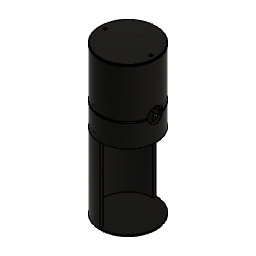
Freshener_Dispenser_Case (Autodesk Fusion 360 design; units mm, degrees)
Autodesk Fusion 360 part; units mm, degrees
note: some values were not read from the file. Chosen so that the rebuilt part matches the saved one: which face or edge a step refers to; which bodies a step acts on; which pieces of a blend or face edit are solid. Set by a fixed rule: which sketch regions a step uses.
(part 1 of 2)
sketch "Sketch1" plane through (0, 0, 0) normal (0, 0, 1) x (1, 0, 0)
  circle A0 centre (0, 0) radius 37.5
  dimension "d1" = 75
  constraint coincident A0.centre origin
  measures "d1" diameter of A0
extrude "Extrude1" add sketch "Sketch1" along normal blind 2 makes body 1
sketch "Sketch2" plane through (0, 0, 2) normal (0, 0, 1) x (-1, 0, 0)
  circle A0 centre (0, 0) radius 37.5
  circle A1 centre (0, 0) radius 33.5
  dimension "d4" = 67
  constraint coincident A0.centre A1.centre
  measures "d4" diameter of A1
extrude "Extrude2" add sketch "Sketch2" along normal blind 196 bodies 1
move_body "Move1" bodies 1 to x (0, 1, 0) y (-1, 0, 0) z (0, 0, 1) at (-0.5, -0.5, 0)
ref_plane "WorkPlane2" through (37, 0, 0) normal (1, 0, 0) x (0, 1, 0)
sketch "Sketch4" plane through (37, 0, 0) normal (1, 0, 0) x (0, 1, 0)
  line L0 (37.676, 2) -> (-39.4371, 2)
  line L1 (-39.4371, 2) -> (-39.4371, 102)
  line L2 (-39.4371, 102) -> (37.676, 102)
  line L3 (37.676, 102) -> (37.676, 2)
  line L4 (37, 0) -> (-38, 0)
  dimension "d14" = 100
  dimension "d15" = 2
  constraint horizontal L0
  constraint vertical L1
  constraint horizontal L2
  constraint vertical L3
  measures "d14" distance of L0.start L2.end
  measures "d15" distance of L0 L4
extrude "Extrude4" cut sketch "Sketch4" against normal blind 37.5 bodies 1
move_body "Move2" bodies 1 to x (1, 0, 0) y (0, 1, 0) z (0, 0, 1) at (0, 0.5, 0)
move_body "Move3" bodies 1 to x (1, 0, 0) y (0, 1, 0) z (0, 0, 1) at (0.5, 0, 0)
sketch "Sketch7" plane through (37, 0, 0) normal (1, 0, 0) x (0, 1, 0)
  circle A0 centre (0, 134) radius 0.25
  circle A1 through (10, 134, 1) (-5, 142.6603, 1) (-5, 125.3397, 1)
  dimension "d33" = 20
sketch "Sketch7 (curves 1 mm off its plane)" plane through (38, 0, 0) normal (1, 0, 0) x (0, 1, 0)
  circle A0 centre (0, 134) radius 10
extrude "Extrude6" cut sketch "Sketch7 (curves 1 mm off its plane)" against normal blind 6 bodies 1
ref_plane "WorkPlane3" through (0, 0, 133.75) normal (0, 0, 1) x (1, 0, 0)
sketch "Sketch6" plane through (0, 0, 133.75) normal (0, 0, 1) x (1, 0, 0)
  circle A0 centre (0, 0) radius 37.5
  spline S0 degree 3 poles (36.345, -9.2353) (36.345, -9.2353) (36.4749, -8.7241) (36.6575, -7.9556) (36.9971, -6.1867) (37.1768, -5.0663) (37.4299, -2.6043) (37.5, -1.2621) (37.5, 1.2621) (37.4299, 2.6043) (37.1768, 5.0663) (36.9971, 6.1867) (36.6575, 7.9556) (36.4749, 8.7241) (36.2151, 9.7465) (36.1421, 10) (36.1421, 10) knots 0 0.378704 0.378704 0.378704 0.378704 0.757408 0.757408 1.136043 1.136043 1.514678 1.514678 1.893313 1.893313 2.271948 2.271948 2.650652 2.650652 3.029356 3.029356 3.029356 3.029356
  line L0 (0, -7) -> (-17, -7)
  line L1 (-17, -7) -> (-17, 7)
  line L2 (-17, 7) -> (0, 7)
  line L3 (36.1439, -9.9936) -> (0, -7)
  line L4 (36.1421, 10) -> (0, 7)
  dimension "d47" = 75
  constraint coincident A0.centre origin
  constraint horizontal L0
  constraint perpendicular L0 L1
  constraint perpendicular L1 L2
  constraint coincident S0.end L4.start
  constraint coincident A0 L3.start
  measures "d47" diameter of A0
extrude "Extrude10" add sketch "Sketch6" against normal blind 2 separate body makes body 2
extrude "Extrude7" cut sketch "Sketch6" against normal blind 2 contours A0 L0 L1 L2 L3 L4 picked at (12.5, 0) bodies 1 2
sketch "Sketch9" plane through (0, 0, 133.75) normal (0, 0, -1) x (-1, 0, 0)
  line L0 (2.5299, 20.125) -> (-2.4701, 20.125)
  line L1 (-2.4701, 20.125) -> (-2.4701, 17.375)
  line L2 (-2.4701, 17.375) -> (2.5299, 17.375)
  line L3 (2.5299, 17.375) -> (2.5299, 20.125)
  line L4 (-2.6701, 17.175) -> (2.7299, 17.175)
  line L5 (2.7299, 17.175) -> (2.7299, 20.325)
  line L6 (2.7299, 20.325) -> (-2.6701, 20.325)
  line L7 (-2.6701, 20.325) -> (-2.6701, 17.175)
  point P0 (-2.4701, 17.375)
  point P1 (2.5299, 17.375)
  point P2 (-2.4701, 20.125)
  point P3 (2.5299, 20.125)
  point P4 (0.0299, 18.75)
  dimension "d43" = 0.2
  constraint coincident P3 L0.start
  constraint coincident P2 L0.end
  constraint coincident P0 L1.end
  constraint coincident P1 L2.end
extrude "Extrude9" cut sketch "Sketch9" along normal blind 5 contours L0 L1 L2 L3 | L4 L5 L6 L7 bodies 1 2
ref_plane "WorkPlane4" through (0, 0, 102) normal (0, 0, 1) x (1, 0, 0)
split "Split1" by plane through (0, 0, 102) normal (0, 0, 1) bodies 1 makes body 3 at (1.8692, 37.4534, 134)
sketch "Sketch10" plane through (0, 0, 102) normal (0, 0, 1) x (-1, 0, 0)
  arc A0 (0, -37.5) -> (0, 37.5) centre (0, 0) ccw
  line L0 (0, 37.5) -> (0, 33.5)
  arc A1 (0, -33.5) -> (0, 33.5) centre (0, 0) ccw
  line L1 (0, -33.5) -> (0, -37.5)
  arc A2 (1.1, -34.5825) -> (1.1, 34.5825) centre (0, 0) ccw
  line L2 (1.1, 36.3834) -> (1.1, 34.5825)
  arc A3 (1.1, -36.3834) -> (1.1, 36.3834) centre (0, 0) ccw
  line L3 (1.1, -34.5825) -> (1.1, -36.3834)
  line L4 (1.3, -34.5756) -> (1.3, -36.3768)
  line L5 (1.3, 36.4) -> (1.3, 34.5756)
  dimension "d90" = 0.2
  dimension "d91" = 0.2
  constraint coincident A2 L4.start
  constraint coincident A3 L4.end
  constraint vertical L4
  constraint vertical L5
  constraint coincident A2 L5.end
  constraint concentric A1 A2
  constraint concentric A0 A3
  measures "d90" distance of L3 L4
  measures "d91" distance of L2 L5
extrude "Extrude11" add sketch "Sketch10" along normal blind 5 contours A2 A3 L4 L5 bodies 1
sketch "Sketch11" plane through (0, 0, 102) normal (0, 0, -1) x (1, 0, 0)
  circle A0 centre (0, 0) radius 33.5
  circle A1 centre (0, 0) radius 37.5
  circle A2 centre (0, 0) radius 36.6
  circle A3 centre (0, 0) radius 34.4
  line L0 (0, 34.4) -> (0, 36.6)
  line L1 (0, -34.4) -> (0, -36.6)
  dimension "d53" = -0.9
  dimension "d54" = 0.9
  constraint coincident A3 L0.start
  constraint coincident A2 L0.end
  constraint vertical L0
  constraint coincident A3 L1.start
  constraint coincident A2 L1.end
  constraint parallel L0 L1
extrude "Extrude12" cut sketch "Sketch11" against normal blind 5.4 contours A2 A3 L0 L1 picked at (-1.8183, -35.7304) bodies 3
ref_plane "WorkPlane5" through (0, 0, 131.75) normal (0, 0, 1) x (1, 0, 0)
split "Split2" by plane through (0, 0, 131.75) normal (0, 0, 1) bodies 3 makes body 4 at (35.2064, 12.9134, 155.3434)
ref_plane "WorkPlane6" through (0, 0, 133.75) normal (0, 0, 1) x (1, 0, 0)
split "Split3" by plane through (0, 0, 133.75) normal (0, 0, 1) bodies 4 makes body 5 at (35.2408, -12.8194, 156.2088)
delete_body "RemoveBody1" bodies 4
sketch "Sketch12" plane through (0, 0, 131.75) normal (0, 0, 1) x (-1, 0, 0)
  line L0 (-32.0517, -9.7436) -> (-36.212, -9.7436)
  arc A0 (-36.212, -9.7436) -> (-36.212, 9.7436) centre (0, 0) ccw
  line L1 (-36.212, 9.7436) -> (-32.0517, 9.7436)
  arc A1 (-32.0517, -9.7436) -> (-32.0517, 9.7436) centre (0, 0) ccw
  arc A2 (-32.8569, -10.8436) -> (-32.8569, 10.8436) centre (0, 0) ccw
  line L2 (-34.7473, 10.8436) -> (-32.8569, 10.8436)
  arc A3 (-34.7473, -10.8436) -> (-34.7473, 10.8436) centre (0, 0) ccw
  line L3 (-32.8569, -10.8436) -> (-34.7473, -10.8436)
  line L4 (36.4, 0) -> (34.6, 0)
  line L5 (-0.0001, -34.6) -> (-0.0001, -36.4)
  line L6 (-0.0001, 36.4) -> (-0.0001, 34.6)
  line L7 (0, 0) -> (25.7387, -25.7387)
  line L8 (0, 0) -> (36.6, 0) construction
  line L9 (0, 0) -> (25.7387, 25.7387)
  line L10 (0, 0) -> (36.6, 0) construction
  line L11 (0, 0) -> (33.6292, -13.9297)
  line L12 (0, 0) -> (36.6, 0) construction
  line L13 (0, 0) -> (33.6292, 13.9297)
  line L14 (0, 0) -> (13.9297, 33.6292)
  line L15 (0, 0) -> (13.9297, -33.6292)
  line L16 (0, 0) -> (36.6, 0) construction
  line L17 (0, 0) -> (-13.9297, 33.6292)
  line L18 (0, 0) -> (36.6, 0) construction
  line L19 (0, 0) -> (-13.9297, -33.6292)
  line L20 (0, 0) -> (-25.8801, -25.8801)
  line L21 (0, 0) -> (36.6, 0) construction
  line L22 (-34.6843, -11.0436) -> (-32.7902, -11.0436)
  line L23 (-25.8797, -25.5969) -> (-24.6069, -24.3241)
  line L24 (13.7447, -33.7052) -> (13.0558, -32.0422)
  line L25 (-13.7387, -33.6908) -> (-13.0558, -32.0422)
  line L26 (33.5522, -14.1142) -> (31.8892, -13.4254)
  line L27 (25.8797, -25.5969) -> (24.6069, -24.3241)
  line L28 (-13.7387, -33.6908) -> (-13.7447, -33.7052)
  dimension "d60" = 45
  dimension "d61" = 45
  dimension "d62" = 22.5
  dimension "d65" = 135
  dimension "d66" = 67.5
  dimension "d67" = 112.5
  dimension "d68" = 45
  dimension "d69" = 135
  dimension "d80" = 0.2
  dimension "d81" = 0.2
  dimension "d82" = 0.2
  dimension "d83" = 0.2
  dimension "d84" = 0.2
  dimension "d85" = 0.2
  constraint midpoint A3 L4.start
  constraint midpoint A2 L4.end
  constraint coincident A2 L5.start
  constraint coincident A3 L5.end
  constraint perpendicular L4 L5
  constraint coincident A3 L6.start
  constraint coincident A2 L6.end
  constraint parallel L5 L6
  constraint horizontal L8
  constraint coincident A0.centre A1.centre
  constraint coincident A3 L7.end
  constraint horizontal L10
  constraint coincident A3 L9.end
  constraint horizontal L12
  constraint coincident A3 L11.end
  constraint coincident A3 L13.end
  constraint coincident A3 L14.end
  constraint horizontal L16
  constraint perpendicular L13 L15
  constraint horizontal L18
  constraint coincident A3 L17.end
  constraint coincident A3 L19.end
  constraint horizontal L21
  constraint coincident A3 L15.end
  constraint coincident A3 L22.start
  constraint coincident A2 L22.end
  constraint parallel L3 L22
  constraint coincident A3 L23.start
  constraint coincident A2 L23.end
  constraint parallel L20 L23
  constraint coincident A3 L24.start
  constraint coincident A2 L24.end
  constraint parallel L15 L24
  constraint coincident A2 L25.end
  constraint parallel L19 L25
  constraint coincident A3 L26.start
  constraint coincident A2 L26.end
  constraint parallel L11 L26
  constraint coincident A3 L27.start
  constraint coincident A2 L27.end
  constraint parallel L7 L27
  constraint coincident A3 L28.end
  constraint parallel L25 L28
  constraint concentric A1 A2
  constraint concentric A0 A3
  measures "d60" angle of L7 L8
  measures "d61" angle of L9 L10
  measures "d62" angle of L11 L12
  measures "d65" angle of L13 L14
  measures "d66" angle of L15 L16
  measures "d67" angle of L17 L18
  measures "d68" angle of L17 L19
  measures "d69" angle of L20 L21
  measures "d80" distance of L3 L22
  measures "d81" distance of L20 L23
  measures "d82" distance of L19 L25
  measures "d83" distance of L15 L24
  measures "d84" distance of L11 L26
  measures "d85" distance of L7 L27
extrude "Extrude13" add sketch "Sketch12" along normal blind 7 contours A2 A3 L22 L23 | A2 A3 L5 L25 L28 | A2 A3 L5 L24 | A2 A3 L26 L27 bodies 3
mirror "Mirror1" about plane through (0, 0, 0) normal (0, 1, 0) of "Extrude13"
sketch "Sketch13" plane through (0, 0, 133.75) normal (0, 0, 1) x (-1, 0, 0)
  line L0 (2.7299, -20.325) -> (-2.6701, -20.325)
  line L1 (-2.6701, -20.325) -> (-2.6701, -17.175)
  line L2 (-2.6701, -17.175) -> (2.7299, -17.175)
  line L3 (2.7299, -17.175) -> (2.7299, -20.325)
  line L4 (0, -7) -> (-36.1421, -10)
  arc A0 (-36.1421, -10) -> (-36.1439, 9.9936) centre (0, 0) ccw
  line L5 (-36.1439, 9.9936) -> (0, 7)
  line L6 (0, 7) -> (17, 7)
  line L7 (17, 7) -> (17, -7)
  line L8 (17, -7) -> (0, -7)
  line L9 (0.0372, 7.9) -> (17.9, 7.9)
  line L10 (17.9, 7.9) -> (17.9, -7.9)
  line L11 (17.9, -7.9) -> (0.0373, -7.9)
  line L12 (0.0373, -7.9) -> (-34.9685, -10.8057)
  arc A1 (-34.9685, -10.8057) -> (-34.9704, 10.7995) centre (0, 0) ccw
  line L13 (-34.9704, 10.7995) -> (0.0372, 7.9)
  arc A2 (-33.1543, -9.1733) -> (-33.156, 9.1675) centre (0, 0) ccw
  line L14 (13.9297, 33.6292) -> (13.2408, 31.9662)
  line L15 (-13.2408, 31.9662) -> (-13.9297, 33.6292)
  line L16 (-25.7387, 25.7387) -> (-24.4659, 24.4659)
  line L17 (-32.8569, 10.8436) -> (-34.7473, 10.8436)
  line L18 (24.4659, 24.4659) -> (25.7387, 25.7387)
  line L19 (33.6292, 13.9297) -> (31.9662, 13.2408)
  line L20 (-32.8569, 10.8436) -> (-32.6462, 10.8436)
  line L21 (-34.7473, 10.8436) -> (-34.9568, 10.8436)
  line L22 (-25.7387, 25.7387) -> (-25.8801, 25.8801)
  line L23 (-24.4659, 24.4659) -> (-24.3245, 24.3245)
  line L24 (-13.9297, 33.6292) -> (-14.0062, 33.814)
  line L25 (-13.2408, 31.9662) -> (-13.1643, 31.7815)
  line L26 (13.9297, 33.6292) -> (14.0062, 33.814)
  line L27 (13.2408, 31.9662) -> (13.1643, 31.7815)
  line L28 (25.7387, 25.7387) -> (25.8801, 25.8801)
  line L29 (24.4659, 24.4659) -> (24.3245, 24.3245)
  line L30 (33.6292, 13.9297) -> (33.814, 14.0062)
  line L31 (31.9662, 13.2408) -> (31.7815, 13.1643)
  dimension "d75" = -3.1
  constraint coincident L17.start L20.start
  constraint coincident A2 L20.end
  constraint parallel L17 L20
  constraint coincident L17.end L21.start
  constraint coincident A1 L21.end
  constraint horizontal L21
  constraint coincident L16.start L22.start
  constraint coincident A1 L22.end
  constraint parallel L16 L22
  constraint coincident L16.end L23.start
  constraint coincident A2 L23.end
  constraint parallel L16 L23
  constraint coincident L15.end L24.start
  constraint coincident A1 L24.end
  constraint parallel L15 L24
  constraint coincident L15.start L25.start
  constraint coincident A2 L25.end
  constraint parallel L15 L25
  constraint coincident L14.start L26.start
  constraint coincident A1 L26.end
  constraint parallel L14 L26
  constraint coincident L14.end L27.start
  constraint coincident A2 L27.end
  constraint parallel L14 L27
  constraint coincident L18.end L28.start
  constraint coincident A1 L28.end
  constraint parallel L18 L28
  constraint coincident L18.start L29.start
  constraint coincident A2 L29.end
  constraint parallel L18 L29
  constraint coincident L19.start L30.start
  constraint coincident A1 L30.end
  constraint parallel L19 L30
  constraint coincident L19.end L31.start
  constraint coincident A2 L31.end
  constraint parallel L19 L31
  constraint concentric A0 A1
extrude "Extrude14" cut sketch "Sketch13" against normal blind 2 contours A1 A2 L18 L19 L28 L29 L30 L31 | A1 A2 L14 L15 L24 L25 L26 L27 | A1 A2 L16 L17 L20 L21 L22 L23 bodies 2
mirror "Mirror2" about plane through (0, 0, 0) normal (0, 1, 0) of "Extrude14"
sketch "Sketch14" plane through (0, 0, 133.75) normal (0, 0, -1) x (1, 0, 0)
  line L0 (36.1429, -9.9969) -> (32, -9.9969)
  line L1 (32, -9.9969) -> (32, -9.9121)
  arc A0 (32, 9.9121) -> (32, -9.9121) centre (0, 0) ccw
  line L2 (32, 9.9121) -> (32, 9.9969)
  line L3 (32, 9.9969) -> (36.1429, 9.9969)
  arc A1 (36.1429, 9.9969) -> (36.1429, -9.9969) centre (0, 0) ccw
  line L4 (32.6462, 10.8436) -> (34.9568, 10.8436)
  arc A2 (32.6462, 10.8436) -> (24.3245, 24.3245) centre (0, 0) ccw
  arc A3 (34.9568, 10.8436) -> (25.8801, 25.8801) centre (0, 0) ccw
  line L5 (25.8801, 25.8801) -> (24.3245, 24.3245)
  arc A4 (13.1643, 31.7815) -> (-13.1643, 31.7815) centre (0, 0) ccw
  arc A5 (14.0062, 33.814) -> (-14.0062, 33.814) centre (0, 0) ccw
  line L6 (-14.0062, 33.814) -> (-13.1643, 31.7815)
  line L7 (13.1643, 31.7815) -> (14.0062, 33.814)
  line L8 (-33.814, 14.0062) -> (-31.7815, 13.1643)
  arc A6 (-25.8801, 25.8801) -> (-33.814, 14.0062) centre (0, 0) ccw
  arc A7 (-24.3245, 24.3245) -> (-31.7815, 13.1643) centre (0, 0) ccw
  line L9 (-24.3245, 24.3245) -> (-25.8801, 25.8801)
extrude "Extrude15" cut sketch "Sketch14" against normal blind 5.4 contours L4 A2 A3 L5 | A4 A5 L6 L7 | L8 A6 A7 L9 bodies 5
mirror "Mirror3" about plane through (0, 0, 0) normal (0, 1, 0) of "Extrude15"
sketch "Sketch15" plane through (0, 0, 198) normal (0, 0, 1) x (-1, 0, 0)
  circle A0 centre (0, 0) radius 33.5
  circle A1 centre (0, 0) radius 37.5
extrude "Extrude16" add sketch "Sketch15" along normal blind 2 separate body contours A0 | A1 makes body 6
sketch "Sketch16" plane through (0, 0, 198) normal (0, 0, -1) x (1, 0, 0)
  circle A0 centre (0, 0) radius 37.5
  circle A1 centre (0.2201, -17) radius 0.75
  circle A2 centre (0.2201, -17) radius 1.25
  dimension "d94" = 0.5
extrude "Extrude17" cut sketch "Sketch16" against normal blind 1 contours A1 | A2 bodies 6
sketch "Sketch19" plane through (0, 0, 198) normal (0, 0, 1) x (-1, 0, 0)
  circle A0 centre (0, 0) radius 33.5
  circle A1 centre (0, 0) radius 37.5
  line L0 (33.1246, -5.0014) -> (28.1246, -5.0014)
  line L1 (28.1246, -5.0014) -> (28.1246, 4.9986)
  line L2 (28.1246, 4.9986) -> (33.125, 4.9986)
  line L3 (33.5, -0.0014) -> (28.1246, -0.0014)
  circle A2 centre (30.8123, -0.0014) radius 1.25
  dimension "d105" = 5
  dimension "d106" = 5
  dimension "d107" = 5
  dimension "d110" = 2.5
  constraint coincident A0 L0.start
  constraint horizontal L0
  constraint perpendicular L0 L1
  constraint coincident A0 L2.end
  constraint perpendicular L1 L2
  constraint coincident A0 L3.start
  constraint coincident L1 L3.end
  constraint perpendicular L1 L3
  constraint midpoint L3 A2.centre
  measures "d105" distance of L0.start L0.end
  measures "d106" distance of L0 L3
  measures "d107" distance of L2 L3
  measures "d110" diameter of A2
extrude "Extrude21" add sketch "Sketch19" against normal blind 3 contours A0 L1 L2 L3 A2 | A0 L0 L1 L3 A2 bodies 5
mirror "Mirror6" about plane through (0, 0, 0) normal (1, 0, 0) of "Extrude21"
sketch "Sketch20" plane through (0, 0, 198) normal (0, 0, -1) x (1, 0, 0)
  circle A0 centre (0.2201, -17) radius 1.25
  circle A1 centre (0, 0) radius 37.5
  circle A2 centre (-30.8123, -0.0014) radius 1.25
  circle A3 centre (-30.8123, -0.0014) radius 2
  dimension "d115" = 0.75
extrude "Extrude22" cut sketch "Sketch20" against normal blind 2 contours A2 | A3 bodies 6
mirror "Mirror7" about plane through (0, 0, 0) normal (1, 0, 0) of "Extrude22"
sketch "Sketch21" plane through (0, 0, 133.75) normal (0, 0, 1) x (-1, 0, 0)
  arc A0 (-14.0062, -33.814) -> (14.0062, -33.814) centre (0, 0) ccw
  line L0 (-14.0062, -33.814) -> (-13.1643, -31.7815)
  arc A1 (-13.1643, -31.7815) -> (13.1643, -31.7815) centre (0, 0) ccw
  line L1 (13.1643, -31.7815) -> (14.0062, -33.814)
  arc A2 (-34.9568, -10.8436) -> (-25.8801, -25.8801) centre (0, 0) ccw
  line L2 (-34.9568, -10.8436) -> (-32.6462, -10.8436)
  arc A3 (-32.6462, -10.8436) -> (-24.3245, -24.3245) centre (0, 0) ccw
  line L3 (-24.3245, -24.3245) -> (-25.8801, -25.8801)
  arc A4 (25.8801, -25.8801) -> (33.814, -14.0062) centre (0, 0) ccw
  line L4 (25.8801, -25.8801) -> (24.3245, -24.3245)
  arc A5 (24.3245, -24.3245) -> (31.7815, -13.1643) centre (0, 0) ccw
  line L5 (31.7815, -13.1643) -> (33.814, -14.0062)
  arc A6 (14.0062, 33.814) -> (-14.0062, 33.814) centre (0, 0) ccw
  line L6 (14.0062, 33.814) -> (13.1643, 31.7815)
  arc A7 (13.1643, 31.7815) -> (-13.1643, 31.7815) centre (0, 0) ccw
  line L7 (-13.1643, 31.7815) -> (-14.0062, 33.814)
  arc A8 (-25.8801, 25.8801) -> (-34.9568, 10.8436) centre (0, 0) ccw
  line L8 (-25.8801, 25.8801) -> (-24.3245, 24.3245)
  arc A9 (-24.3245, 24.3245) -> (-32.6462, 10.8436) centre (0, 0) ccw
  line L9 (-32.6462, 10.8436) -> (-34.9568, 10.8436)
  arc A10 (33.814, 14.0062) -> (25.8801, 25.8801) centre (0, 0) ccw
  line L10 (33.814, 14.0062) -> (31.7815, 13.1643)
  arc A11 (31.7815, 13.1643) -> (24.3245, 24.3245) centre (0, 0) ccw
  line L11 (24.3245, 24.3245) -> (25.8801, 25.8801)
  line L12 (2.7299, -20.325) -> (-2.6701, -20.325)
  line L13 (-2.6701, -20.325) -> (-2.6701, -17.175)
  line L14 (-2.6701, -17.175) -> (2.7299, -17.175)
  line L15 (2.7299, -17.175) -> (2.7299, -20.325)
  line L16 (0, -7) -> (-36.1421, -10)
  arc A12 (-36.1421, -10) -> (-36.1439, 9.9936) centre (0, 0) ccw
  line L17 (-36.1439, 9.9936) -> (0, 7)
  line L18 (0, 7) -> (17, 7)
  line L19 (17, 7) -> (17, -7)
  line L20 (17, -7) -> (0, -7)
  line L21 (-36.0448, 11.1895) -> (0.0496, 8.2)
  line L22 (0.0496, 8.2) -> (18.2, 8.2)
  line L23 (18.2, 8.2) -> (18.2, -8.2)
  line L24 (18.2, -8.2) -> (0.0497, -8.2)
  line L25 (0.0497, -8.2) -> (-36.0428, -11.1959)
  line L26 (-31.578, 9.6154) -> (-31.1283, 10.7823)
  spline S0 degree 3 poles (-32.0517, 9.7436) (-32.0896, 9.619) (-32.1408, 9.4481) (-32.3488, 8.7229) (-32.5544, 7.9547) (-32.936, 6.1877) (-33.1376, 5.0683) (-33.4214, 2.6067) (-33.5, 1.2638) (-33.5, -1.2638) (-33.4214, -2.6067) (-33.1376, -5.0683) (-32.936, -6.1877) (-32.5544, -7.9547) (-32.3488, -8.7229) (-32.1408, -9.4481) (-32.0896, -9.619) (-32.0517, -9.7436) knots 0.220731 0.220731 0.220731 0.220731 0.37925 0.37925 0.7585 0.7585 1.137639 1.137639 1.516778 1.516778 1.895917 1.895917 2.275056 2.275056 2.654306 2.654306 2.812825 2.812825 2.812825 2.812825
  line L27 (11.9299, -8.2) -> (11.9299, -7)
  line L28 (11.2799, -8) -> (11.2799, -26)
  line L29 (-11.8701, -9.1894) -> (-11.8701, -7.9853)
  line L30 (-11.2201, -8.25) -> (-11.2201, -13.9459)
  line L31 (-35.7961, -11.1754) -> (-36.1421, -10)
  line L32 (-31.2057, -10.7944) -> (-31.5517, -9.619)
  point P0 (-32.078, 9.6568)
  point P1 (11.2799, -8.2)
  point P2 (-11.2201, -9.1355)
  dimension "d120" = -1.2
  dimension "d121" = 0.5
  dimension "d124" = 0.65
  dimension "d125" = 0.65
  dimension "d126" = 0.5
  constraint coincident L17 L26.start
  constraint coincident L21 L26.end
  constraint coincident S0 P0
  constraint coincident L17 P0
  constraint coincident L24 L27.start
  constraint coincident L20 L27.end
  constraint perpendicular L20 L27
  constraint coincident L28 P1
  constraint coincident L24 P1
  constraint coincident L25 L29.start
  constraint coincident L16 L29.end
  constraint vertical L29
  constraint coincident L30 P2
  constraint coincident L25 P2
  constraint coincident L25 L31.start
  constraint coincident A12 L31.start
  constraint coincident L16.end A12.start
  constraint coincident L25 L32.start
  constraint coincident L16 L32.end
  constraint parallel L31 L32
  measures "d121" horizontal distance of L26.start P0
  measures "d124" distance of L27.start P1
  measures "d125" horizontal distance of L29.start P2
  measures "d126" distance of S0.end L32.end
extrude "Extrude23" add sketch "Sketch21" along normal blind 25 contours L16 L25 L29 L32 | L17 L18 L19 L20 L21 L22 L23 L24 L26 L27 bodies 2
sketch "Sketch22" plane through (0, 0, 158.75) normal (0, 0, 1) x (-1, 0, 0)
  line L0 (-31.578, 9.6154) -> (0, 7)
  line L1 (0, 7) -> (17, 7)
  line L2 (17, 7) -> (17, -7)
  line L3 (17, -7) -> (11.9299, -7)
  line L4 (11.9299, -7) -> (11.9299, -8.2)
  line L5 (11.9299, -8.2) -> (18.2, -8.2)
  line L6 (18.2, -8.2) -> (18.2, 8.2)
  line L7 (18.2, 8.2) -> (0.0496, 8.2)
  line L8 (0.0496, 8.2) -> (-31.1283, 10.7823)
  line L9 (-31.1283, 10.7823) -> (-31.578, 9.6154)
  line L10 (18.2, -8.2) -> (18.2, 8.2)
  line L11 (18.2, 8.2) -> (0.0496, 8.2)
  line L12 (-31.1283, 10.7823) -> (0.0496, 8.2)
  line L13 (18.2, -8.2) -> (11.9299, -8.2)
  line L14 (-31.2057, -10.7944) -> (-11.8701, -9.1894)
  spline S0 degree 5 poles (-31.2057, -10.7944) (-31.3407, -10.3619) (-31.5987, -9.4971) (-31.9499, -8.2001) (-32.3455, -6.4712) (-32.7107, -4.311) (-32.9348, -2.1517) (-33.0065, 0.0065) (-32.9195, 2.1636) (-32.6799, 4.3197) (-32.2993, 6.4748) (-31.8912, 8.1982) (-31.5306, 9.4904) (-31.2664, 10.3517) (-31.1283, 10.7823) knots 0 0 0 0 0 0 0.1 0.2 0.3 0.4 0.5 0.6 0.7 0.8 0.9 1 1 1 1 1 1
  line L15 (11.9299, -8.2) -> (11.9299, -7)
  line L16 (11.9299, -7) -> (-11.8701, -7)
  line L17 (-11.8701, -7) -> (-11.8701, -9.1894)
  point P0 (-31.2057, -10.7944)
  point P1 (-11.8701, -9.1894)
  point P2 (-32.9669, 0.0108)
  constraint coincident L5.end L6.start
  constraint coincident L6.end L7.start
  constraint coincident L7.end L8.start
  constraint coincident L8.end L9.start
  constraint coincident L4.end L5.start
  constraint coincident P0 L14.start
  constraint coincident P1 L14.end
  constraint coincident L3.end L4.start
  constraint perpendicular L15 L16
  constraint parallel L15 L17
extrude "Extrude24" add sketch "Sketch22" along normal blind 1.2 separate body contours L0 L1 L2 L3 L4 L5 L6 L7 L8 L10 L11 L12 L13 S0 L15 | L0 L1 L2 L3 L14 S0 L16 L17 makes body 7
sketch "Sketch23" plane through (0, 0, 159.95) normal (0, 0, 1) x (-1, 0, 0)
  line L0 (18.2, -8.2) -> (18.2, 8.2)
  line L1 (18.2, 8.2) -> (0.0496, 8.2)
  line L2 (0.0496, 8.2) -> (-31.1283, 10.7823)
  spline S0 degree 5 poles (-31.1283, 10.7823) (-31.2664, 10.3517) (-31.5306, 9.4904) (-31.8912, 8.1982) (-32.2993, 6.4748) (-32.6799, 4.3197) (-32.9195, 2.1636) (-33.0065, 0.0065) (-32.9348, -2.1517) (-32.7107, -4.311) (-32.3455, -6.4712) (-31.9499, -8.2001) (-31.5987, -9.4971) (-31.3407, -10.3619) (-31.2057, -10.7944) knots -1 -1 -1 -1 -1 -1 -0.9 -0.8 -0.7 -0.6 -0.5 -0.4 -0.3 -0.2 -0.1 0 0 0 0 0 0
  line L3 (-31.2057, -10.7944) -> (-11.8701, -9.1894)
  line L4 (-11.8701, -9.1894) -> (-11.8701, -7)
  line L5 (-11.8701, -7) -> (11.9299, -7)
  line L6 (11.9299, -7) -> (11.9299, -8.2)
  line L7 (11.9299, -8.2) -> (18.2, -8.2)
  line L8 (12.4345, 7.3206) -> (12.4345, 8.2)
  line L9 (10.437, 7.3206) -> (10.437, 8.2)
  line L10 (9.937, 7.3206) -> (9.937, 8.2)
  line L11 (9.937, 7.3206) -> (9.937, -5.3794)
  line L12 (9.937, -5.3794) -> (9.937, -6.831)
  line L13 (12.9345, -5.3794) -> (12.9345, 7.3206)
  line L14 (12.9345, 7.3206) -> (12.9345, 8.2)
  line L15 (9.937, -6.831) -> (9.937, -7)
  line L16 (-6.5642, -4.356) -> (-4.5642, -4.356)
  line L17 (-6.5642, -3.106) -> (-4.5642, -3.106)
  line L18 (-4.5642, -4.356) -> (-3.9392, -4.356)
  line L19 (-3.9392, -4.356) -> (-3.9392, -3.106)
  line L20 (-3.9392, -3.106) -> (-4.5642, -3.106)
  line L21 (-6.5642, -3.106) -> (-7.1892, -3.106)
  line L22 (-7.1892, -3.106) -> (-7.1892, -4.356)
  line L23 (-7.1892, -4.356) -> (-6.5642, -4.356)
  line L24 (-3.1892, -5.106) -> (-3.1892, -2.356)
  line L25 (-3.1892, -2.356) -> (-4.5642, -2.356)
  line L26 (-6.5642, -2.356) -> (-4.5642, -2.356)
  line L27 (-6.5642, -2.356) -> (-7.9392, -2.356)
  line L28 (-7.9392, -2.356) -> (-7.9392, -5.106)
  line L29 (-7.9392, -5.106) -> (-6.5642, -5.106)
  line L30 (-6.5642, -5.106) -> (-4.5642, -5.106)
  line L31 (-4.5642, -5.106) -> (-3.1892, -5.106)
  line L32 (7.6451, 4.4702) -> (7.6451, 8.2)
  line L33 (7.6451, 4.4702) -> (6.5189, 4.4702)
  line L34 (6.5189, 4.4702) -> (6.4807, 8.2)
  line L35 (5.7765, 3.7202) -> (5.7308, 8.1923)
  line L36 (8.3951, 3.7202) -> (5.7765, 3.7202)
  line L37 (8.3951, 3.7202) -> (8.3951, 8.2)
  line L38 (8.3951, 8.2) -> (7.6451, 8.2)
  line L39 (8.3951, 8.2) -> (7.6451, 8.2)
  line L40 (5.7308, 8.1923) -> (5.7308, 8.2)
  line L41 (6.4807, 8.2) -> (5.7308, 8.2)
  circle A0 centre (-28.0642, 7.769) radius 1.5
  circle A1 centre (-28.0642, -5.731) radius 1.5
  circle A2 centre (-28.0642, 7.769) radius 0.75
  circle A3 centre (-28.0642, -5.731) radius 0.75
  dimension "d132" = 0.75
  dimension "d133" = -0.75
  dimension "d136" = 1.5
  dimension "d137" = 1.5
  constraint coincident L1 L8.end
  constraint perpendicular L1 L8
  constraint coincident L1 L9.end
  constraint perpendicular L1 L9
  constraint coincident L5 L15.end
  constraint perpendicular L5 L15
  constraint horizontal L16
  constraint parallel L16 L17
  constraint parallel L16 L18
  constraint perpendicular L17 L19
  constraint perpendicular L19 L20
  constraint parallel L17 L21
  constraint perpendicular L16 L22
  constraint perpendicular L22 L23
  constraint coincident L1 L32.end
  constraint perpendicular L1 L32
  constraint perpendicular L32 L33
  constraint coincident L1 L34.end
  constraint perpendicular L32 L38
  constraint coincident L1 L40.end
  constraint perpendicular L1 L40
  constraint concentric A0 A2
  constraint concentric A1 A3
  measures "d136" diameter of A2
  measures "d137" diameter of A3
extrude "Extrude25" cut sketch "Sketch23" against normal blind 1.2 contours L0 L1 L5 L6 L7 L10 L11 L12 L15 bodies 7
extrude "Extrude26" cut sketch "Sketch23" against normal blind 1.2 contours L1 L32 L33 L34 L35 L36 L37 L38 L39 L40 L41 | L1 L32 L33 L34 | L16 L17 L18 L19 L20 L21 L22 L23 | L24 L25 L26 L27 L28 L29 L30 L31 | A2 | A3 bodies 7
sketch "Sketch24" plane through (0, 0, 133.75) normal (0, 0, 1) x (-1, 0, 0)
  line L0 (-31.2057, -10.7944) -> (-31.5517, -9.619)
  line L1 (-31.5517, -9.619) -> (-36.1421, -10)
  arc A0 (-36.1421, -10) -> (-36.1439, 9.9936) centre (0, 0) ccw
  line L2 (-36.1439, 9.9936) -> (-31.578, 9.6154)
  line L3 (-31.578, 9.6154) -> (-31.1283, 10.7823)
  line L4 (-31.1283, 10.7823) -> (0.0496, 8.2)
  line L5 (0.0496, 8.2) -> (18.2, 8.2)
  line L6 (18.2, 8.2) -> (18.2, -8.2)
  line L7 (18.2, -8.2) -> (11.9299, -8.2)
  line L8 (11.9299, -8.2) -> (11.9299, -7)
  line L9 (11.9299, -7) -> (0, -7)
  line L10 (0, -7) -> (-11.8701, -7.9853)
  line L11 (-11.8701, -7.9853) -> (-11.8701, -9.1894)
  line L12 (-11.8701, -9.1894) -> (-31.2057, -10.7944)
  arc A1 (-14.0062, -33.814) -> (14.0062, -33.814) centre (0, 0) ccw
  line L13 (-14.0062, -33.814) -> (-13.1643, -31.7815)
  arc A2 (-13.1643, -31.7815) -> (13.1643, -31.7815) centre (0, 0) ccw
  line L14 (13.1643, -31.7815) -> (14.0062, -33.814)
  arc A3 (-34.9568, -10.8436) -> (-25.8801, -25.8801) centre (0, 0) ccw
  line L15 (-34.9568, -10.8436) -> (-32.6462, -10.8436)
  arc A4 (-32.6462, -10.8436) -> (-24.3245, -24.3245) centre (0, 0) ccw
  line L16 (-24.3245, -24.3245) -> (-25.8801, -25.8801)
  arc A5 (25.8801, -25.8801) -> (33.814, -14.0062) centre (0, 0) ccw
  line L17 (25.8801, -25.8801) -> (24.3245, -24.3245)
  arc A6 (24.3245, -24.3245) -> (31.7815, -13.1643) centre (0, 0) ccw
  line L18 (31.7815, -13.1643) -> (33.814, -14.0062)
  arc A7 (14.0062, 33.814) -> (-14.0062, 33.814) centre (0, 0) ccw
  line L19 (14.0062, 33.814) -> (13.1643, 31.7815)
  arc A8 (13.1643, 31.7815) -> (-13.1643, 31.7815) centre (0, 0) ccw
  line L20 (-13.1643, 31.7815) -> (-14.0062, 33.814)
  arc A9 (-25.8801, 25.8801) -> (-34.9568, 10.8436) centre (0, 0) ccw
  line L21 (-25.8801, 25.8801) -> (-24.3245, 24.3245)
  arc A10 (-24.3245, 24.3245) -> (-32.6462, 10.8436) centre (0, 0) ccw
  line L22 (-32.6462, 10.8436) -> (-34.9568, 10.8436)
  arc A11 (33.814, 14.0062) -> (25.8801, 25.8801) centre (0, 0) ccw
  line L23 (33.814, 14.0062) -> (31.7815, 13.1643)
  arc A12 (31.7815, 13.1643) -> (24.3245, 24.3245) centre (0, 0) ccw
  line L24 (24.3245, 24.3245) -> (25.8801, 25.8801)
  line L25 (2.7299, -20.325) -> (-2.6701, -20.325)
  line L26 (-2.6701, -20.325) -> (-2.6701, -17.175)
  line L27 (-2.6701, -17.175) -> (2.7299, -17.175)
  line L28 (2.7299, -17.175) -> (2.7299, -20.325)
  circle A13 centre (20.8, 11.2) radius 1
  circle A14 centre (-20.5, 11.2) radius 1
  circle A15 centre (20.8, 11.2) radius 0.75
  circle A16 centre (-20.5, 11.2) radius 0.75
  ellipse E0 centre (-17.6329, 26.63) end of major axis (-17.6329, 25.7781) minor radius 0.8519
  ellipse E1 centre (17.9271, 26.63) end of major axis (17.9271, 25.7781) minor radius 0.8519
  line L29 (17.9271, 26.63) -> (-17.6329, 26.63)
  line L30 (17.9271, 26.63) -> (17.9271, 25.7781)
  line L31 (17.9271, 26.63) -> (17.9271, 27.4819)
  line L32 (17.9271, 25.7781) -> (-17.6329, 25.7781)
  line L33 (17.9271, 27.4819) -> (-17.6329, 27.4819)
  line L34 (17.9271, 26.63) -> (18.779, 26.63)
  line L35 (18.779, 26.63) -> (18.779, 25.7781)
  line L36 (18.779, 25.7781) -> (17.9271, 25.7781)
  line L37 (17.9271, 27.4819) -> (18.779, 27.4819)
  line L38 (18.779, 27.4819) -> (18.779, 26.63)
  line L39 (-17.6329, 26.63) -> (-18.4848, 26.63)
  line L40 (-18.4848, 26.63) -> (-18.4848, 25.7781)
  line L41 (-18.4848, 25.7781) -> (-17.6329, 25.7781)
  line L42 (-18.4848, 26.63) -> (-18.4848, 27.4819)
  line L43 (-18.4848, 27.4819) -> (-17.6329, 27.4819)
  line L44 (19.279, 26.63) -> (19.279, 25.2781)
  line L45 (19.279, 25.2781) -> (17.9271, 25.2781)
  line L46 (17.9271, 25.2781) -> (-17.6329, 25.2781)
  line L47 (-18.9848, 25.2781) -> (-17.6329, 25.2781)
  line L48 (-18.9848, 26.63) -> (-18.9848, 25.2781)
  line L49 (-18.9848, 26.63) -> (-18.9848, 27.9819)
  line L50 (-18.9848, 27.9819) -> (-17.6329, 27.9819)
  line L51 (17.9271, 27.9819) -> (-17.6329, 27.9819)
  line L52 (17.9271, 27.9819) -> (19.279, 27.9819)
  line L53 (19.279, 27.9819) -> (19.279, 26.63)
  dimension "d138" = 1.5
  dimension "d139" = 1.5
  dimension "d142" = -0.5
  constraint concentric A13 A15
  constraint concentric A14 A16
  constraint coincident E1.centre L29.start
  constraint coincident E0.centre L29.end
  constraint coincident E1 L30.end
  constraint perpendicular L29 L30
  constraint coincident E1 L31.end
  constraint perpendicular L29 L31
  constraint coincident E0 L32.end
  constraint perpendicular L30 L32
  constraint coincident E0 L33.end
  constraint tangent E1 L33
  constraint coincident E1 L34.end
  constraint parallel L29 L34
  constraint perpendicular L29 L35
  constraint perpendicular L35 L36
  constraint perpendicular L31 L37
  constraint perpendicular L37 L38
  constraint coincident E0 L39.end
  constraint perpendicular L38 L39
  constraint perpendicular L32 L40
  constraint perpendicular L40 L41
  constraint perpendicular L33 L42
  constraint perpendicular L42 L43
  measures "d138" diameter of A15
  measures "d139" diameter of A16
extrude "Extrude27" cut sketch "Sketch24" against normal blind 2 contours A15 | A16 bodies 2
extrude "Extrude28" add sketch "Sketch24" along normal blind 1.5 contours L44 L45 L46 L47 L48 L49 L50 L51 L52 L53 bodies 2
ref_plane "WorkPlane8" through (0, -33.5, 0) normal (0, 1, 0) x (0, 0, 1)
sketch "Sketch27" plane through (0, -33.5, 0) normal (0, 1, 0) x (1, 0, 0)
  circle A0 centre (8.8696, -178.6636) radius 1.75
  circle A1 centre (8.8696, -178.6636) radius 2.25
  dimension "d154" = 0.5
extrude "Extrude31" add sketch "Sketch27" along normal blind 3.25 contours A0 | A1 bodies 5
mirror "Mirror9" about plane through (0, 0, 0) normal (1, 0, 0) of "Extrude31"
sketch "Sketch28" plane through (0, -30.25, 0) normal (0, 1, 0) x (-1, 0, 0)
  circle A0 centre (-8.8696, 178.6636) radius 2.25
  circle A1 centre (-8.8696, 178.6636) radius 0.875
  dimension "d160" = 1.75
  constraint concentric A0 A1
  measures "d160" diameter of A1
extrude "Extrude32" cut sketch "Sketch28" against normal blind 4 contours A1 bodies 5
fillet "Fillet1" radius 0.5 2 edges at (13.5606, -34.9623, 0) (34.9623, 13.5606, 200) on bodies 1 6
sketch "Sketch29" plane through (0, 0, 133.75) normal (0, 0, 1) x (-1, 0, 0)
  line L0 (2.7299, -20.325) -> (-2.6701, -20.325)
  line L1 (-2.6701, -20.325) -> (-2.6701, -17.175)
  line L2 (-2.6701, -17.175) -> (2.7299, -17.175)
  line L3 (2.7299, -17.175) -> (2.7299, -20.325)
  arc A0 (33.814, 14.0062) -> (25.8801, 25.8801) centre (0, 0) ccw
  line L4 (33.814, 14.0062) -> (31.7815, 13.1643)
  arc A1 (31.7815, 13.1643) -> (24.3245, 24.3245) centre (0, 0) ccw
  line L5 (24.3245, 24.3245) -> (25.8801, 25.8801)
  arc A2 (-25.8801, 25.8801) -> (-34.9568, 10.8436) centre (0, 0) ccw
  line L6 (-25.8801, 25.8801) -> (-24.3245, 24.3245)
  arc A3 (-24.3245, 24.3245) -> (-32.6462, 10.8436) centre (0, 0) ccw
  line L7 (-32.6462, 10.8436) -> (-34.9568, 10.8436)
  arc A4 (14.0062, 33.814) -> (-14.0062, 33.814) centre (0, 0) ccw
  line L8 (14.0062, 33.814) -> (13.1643, 31.7815)
  arc A5 (13.1643, 31.7815) -> (-13.1643, 31.7815) centre (0, 0) ccw
  line L9 (-13.1643, 31.7815) -> (-14.0062, 33.814)
  arc A6 (25.8801, -25.8801) -> (33.814, -14.0062) centre (0, 0) ccw
  line L10 (25.8801, -25.8801) -> (24.3245, -24.3245)
  arc A7 (24.3245, -24.3245) -> (31.7815, -13.1643) centre (0, 0) ccw
  line L11 (31.7815, -13.1643) -> (33.814, -14.0062)
  arc A8 (-34.9568, -10.8436) -> (-25.8801, -25.8801) centre (0, 0) ccw
  line L12 (-34.9568, -10.8436) -> (-32.6462, -10.8436)
  arc A9 (-32.6462, -10.8436) -> (-24.3245, -24.3245) centre (0, 0) ccw
  line L13 (-24.3245, -24.3245) -> (-25.8801, -25.8801)
  arc A10 (-14.0062, -33.814) -> (14.0062, -33.814) centre (0, 0) ccw
  line L14 (-14.0062, -33.814) -> (-13.1643, -31.7815)
  arc A11 (-13.1643, -31.7815) -> (13.1643, -31.7815) centre (0, 0) ccw
  line L15 (13.1643, -31.7815) -> (14.0062, -33.814)
  line L16 (-31.2057, -10.7944) -> (-31.5517, -9.619)
  line L17 (-31.5517, -9.619) -> (-36.1421, -10)
  arc A12 (-36.1421, -10) -> (-36.1439, 9.9936) centre (0, 0) ccw
  line L18 (-36.1439, 9.9936) -> (-31.578, 9.6154)
  line L19 (-31.578, 9.6154) -> (-31.1283, 10.7823)
  line L20 (-31.1283, 10.7823) -> (0.0496, 8.2)
  line L21 (0.0496, 8.2) -> (18.2, 8.2)
  line L22 (18.2, 8.2) -> (18.2, -8.2)
  line L23 (18.2, -8.2) -> (11.9299, -8.2)
  line L24 (11.9299, -8.2) -> (11.9299, -7)
  line L25 (11.9299, -7) -> (0, -7)
  line L26 (0, -7) -> (-11.8701, -7.9853)
  line L27 (-11.8701, -7.9853) -> (-11.8701, -9.1894)
  line L28 (-11.8701, -9.1894) -> (-31.2057, -10.7944)
  circle A13 centre (-20.5, 11.2) radius 0.75
  circle A14 centre (20.8, 11.2) radius 0.75
  line L29 (19.279, 27.9819) -> (19.279, 25.2781)
  line L30 (19.279, 25.2781) -> (-18.9848, 25.2781)
  line L31 (-18.9848, 25.2781) -> (-18.9848, 27.9819)
  line L32 (-18.9848, 27.9819) -> (19.279, 27.9819)
  line L33 (-11.2201, -9.075) -> (-11.2201, -14.7709)
  line L34 (-11.2201, -26.825) -> (-11.2201, -22.0709)
  arc A15 (-11.2201, -26.825) -> (-10.9701, -27.075) centre (-10.9701, -26.825) ccw
  line L35 (-10.9701, -27.075) -> (11.0299, -27.075)
  arc A16 (11.0299, -27.075) -> (11.2799, -26.825) centre (11.0299, -26.825) ccw
  line L36 (11.2799, -22.0709) -> (11.2799, -26.825)
  line L37 (11.2799, -14.7709) -> (11.2799, -9.075)
  line L38 (11.2799, -22.0709) -> (11.2799, -14.7709)
  line L39 (-11.2201, -22.0709) -> (-11.2201, -14.7709)
  line L40 (-11.4201, -9.075) -> (-11.4201, -14.7709)
  line L41 (-11.4201, -22.0709) -> (-11.4201, -14.7709)
  line L42 (-11.4201, -26.825) -> (-11.4201, -22.0709)
  arc A17 (-11.4201, -26.825) -> (-10.9701, -27.275) centre (-10.9701, -26.825) ccw
  line L43 (-10.9701, -27.275) -> (11.0299, -27.275)
  arc A18 (11.0299, -27.275) -> (11.4799, -26.825) centre (11.0299, -26.825) ccw
  line L44 (11.4799, -22.0709) -> (11.4799, -26.825)
  line L45 (11.4799, -22.0709) -> (11.4799, -14.7709)
  line L46 (11.4799, -14.7709) -> (11.4799, -9.075)
  line L47 (-12.6201, -9.075) -> (-12.6201, -14.7709)
  line L48 (-12.6201, -22.0709) -> (-12.6201, -14.7709)
  line L49 (-12.6201, -26.825) -> (-12.6201, -22.0709)
  arc A19 (-12.6201, -26.825) -> (-10.9701, -28.475) centre (-10.9701, -26.825) ccw
  line L50 (-10.9701, -28.475) -> (11.0299, -28.475)
  arc A20 (11.0299, -28.475) -> (12.6799, -26.825) centre (11.0299, -26.825) ccw
  line L51 (12.6799, -22.0709) -> (12.6799, -26.825)
  line L52 (12.6799, -22.0709) -> (12.6799, -14.7709)
  line L53 (12.6799, -14.7709) -> (12.6799, -9.075)
  line L54 (-11.4201, -9.075) -> (-11.4201, -7.9479)
  line L55 (11.4799, -9.075) -> (11.4799, -7)
  line L56 (12.6799, -9.075) -> (12.6799, -8.2)
  dimension "d169" = 0.2
  dimension "d170" = 1.4
  constraint coincident L36.start L38.start
  constraint coincident L37.start L38.end
  constraint coincident L34.end L39.start
  constraint coincident L33.end L39.end
  constraint coincident L26 L54.end
  constraint parallel L40 L54
  constraint coincident L25 L55.end
  constraint perpendicular L25 L55
  constraint coincident L23 L56.end
  constraint perpendicular L23 L56
extrude "Extrude33" add sketch "Sketch29" along normal blind 15 contours L23 L24 L25 L26 L27 L28 L40 L41 L42 A17 L43 A18 L44 L45 L46 L47 L48 L49 A19 L50 A20 L51 L52 L53 L54 L55 L56 bodies 2
sketch "Sketch30" plane through (0, 0, 148.75) normal (0, 0, 1) x (-1, 0, 0)
  line L0 (12.6799, -26.825) -> (12.6799, -8.2)
  line L1 (12.6799, -8.2) -> (11.9299, -8.2)
  line L2 (11.9299, -8.2) -> (11.9299, -7)
  line L3 (11.9299, -7) -> (11.4799, -7)
  line L4 (11.4799, -7) -> (11.4799, -26.825)
  arc A0 (11.0299, -27.275) -> (11.4799, -26.825) centre (11.0299, -26.825) ccw
  line L5 (11.0299, -27.275) -> (-10.9701, -27.275)
  arc A1 (-11.4201, -26.825) -> (-10.9701, -27.275) centre (-10.9701, -26.825) ccw
  line L6 (-11.4201, -26.825) -> (-11.4201, -7.9479)
  line L7 (-11.4201, -7.9479) -> (-11.8701, -7.9853)
  line L8 (-11.8701, -7.9853) -> (-11.8701, -9.1894)
  line L9 (-11.8701, -9.1894) -> (-12.6201, -9.2517)
  line L10 (-12.6201, -9.2517) -> (-12.6201, -26.825)
  arc A2 (-12.6201, -26.825) -> (-10.9701, -28.475) centre (-10.9701, -26.825) ccw
  line L11 (-10.9701, -28.475) -> (11.0299, -28.475)
  arc A3 (11.0299, -28.475) -> (12.6799, -26.825) centre (11.0299, -26.825) ccw
  line L12 (-11.8701, -9.1894) -> (-11.4201, -9.1894)
  line L13 (11.9299, -8.2) -> (11.4799, -8.2)
  constraint coincident L8.end L9.start
  constraint coincident L6 L12.end
  constraint perpendicular L6 L12
  constraint coincident L1.end L2.start
  constraint coincident L4 L13.end
  constraint perpendicular L4 L13
extrude "Extrude34" add sketch "Sketch30" along normal blind 10 contours L2 L3 L4 L13 | L6 L7 L8 L12 bodies 2
sketch "Sketch31" plane through (0, 0, 133.75) normal (0, 0, 1) x (-1, 0, 0)
  line L0 (-11.4201, -7.9479) -> (-11.4201, -26.825)
  arc A0 (-11.4201, -26.825) -> (-10.9701, -27.275) centre (-10.9701, -26.825) ccw
  line L1 (-10.9701, -27.275) -> (11.0299, -27.275)
  arc A1 (11.0299, -27.275) -> (11.4799, -26.825) centre (11.0299, -26.825) ccw
  line L2 (11.4799, -26.825) -> (11.4799, -7)
  line L3 (11.4799, -7) -> (0, -7)
  line L4 (0, -7) -> (-11.4201, -7.9479)
  line L5 (2.7299, -20.325) -> (-2.6701, -20.325)
  line L6 (-2.6701, -20.325) -> (-2.6701, -17.175)
  line L7 (-2.6701, -17.175) -> (2.7299, -17.175)
  line L8 (2.7299, -17.175) -> (2.7299, -20.325)
  line L9 (11.4799, -5.8) -> (-0.0497, -5.8)
  line L10 (-0.0497, -5.8) -> (-11.5194, -6.752)
  line L11 (-11.5194, -6.752) -> (-11.4201, -7.9479)
  line L12 (11.4799, -5.8) -> (11.4799, -7)
  dimension "d175" = 1.2
  constraint coincident L0.start L4.end
  constraint perpendicular L4 L11
  constraint coincident L2.end L3.start
  constraint perpendicular L3 L12
extrude "Extrude35" add sketch "Sketch31" against normal blind 2 contours L3 L4 L9 L10 L11 L12 bodies 2
extrude "Extrude36" add sketch "Sketch31" along normal blind 7 contours L3 L4 L9 L10 L11 L12 bodies 2 3
extrude "Extrude37" add 1 faces at (11.4863, 7.1507, 135.4167) along direction (0.996573, 0.082721, 0) blind 5 on bodies 2 bodies 2
extrude "Extrude38" add 1 faces at (-11.4799, 6.2, 135.4167) along direction (-1, 0, 0) blind 6 on bodies 2 bodies 2
extrude "Extrude39" add 1 faces at (0.4423, 17.8521, 199) along direction (0, 0, -1) blind 1 on bodies 6 bodies 6
sketch "Sketch32" plane through (0, 0, 198) normal (0, 0, -1) x (1, 0, 0)
  circle A0 centre (30.8123, -0.0014) radius 2
  circle A1 centre (-30.8123, -0.0014) radius 2
  circle A2 centre (0, 0) radius 37.5
  circle A3 centre (0.2201, -17.825) radius 0.75
  circle A4 centre (0.2201, -17.825) radius 1.75
  arc A5 (11.2201, -14.7709) -> (6.2201, -9.7709) centre (6.2201, -14.7709) ccw
  line L0 (-6.2799, -9.7709) -> (6.2201, -9.7709)
  arc A6 (-6.2799, -9.7709) -> (-11.2799, -14.7709) centre (-6.2799, -14.7709) ccw
  arc A7 (-11.2799, -22.0715) -> (-8.5299, -26.536) centre (-6.2799, -22.0709) ccw
  arc A8 (8.4701, -26.536) -> (11.2201, -22.0715) centre (6.2201, -22.0709) ccw
  line L1 (3.9701, -28.0709) -> (-4.0299, -28.0709)
  line L2 (11.2201, -14.7709) -> (11.2201, -22.0715)
  line L3 (-6.2799, -9.4709) -> (6.2201, -9.4709)
  arc A9 (11.5201, -14.7709) -> (6.2201, -9.4709) centre (6.2201, -14.7709) ccw
  line L4 (11.5201, -14.7709) -> (11.5201, -22.0715)
  arc A10 (8.5863, -26.8133) -> (11.5201, -22.0715) centre (6.2201, -22.0709) ccw
  line L5 (4.0199, -28.3709) -> (-4.0796, -28.3709)
  arc A11 (-11.5799, -22.0715) -> (-8.6461, -26.8133) centre (-6.2799, -22.0709) ccw
  arc A12 (-6.2799, -9.4709) -> (-11.5799, -14.7709) centre (-6.2799, -14.7709) ccw
  arc A13 (-6.2799, -8.5709) -> (-12.4799, -14.7709) centre (-6.2799, -14.7709) ccw
  arc A14 (-12.4799, -22.0715) -> (-8.9915, -27.6464) centre (-6.2799, -22.0709) ccw
  line L6 (4.1692, -29.2709) -> (-4.2289, -29.2709)
  arc A15 (8.9318, -27.6464) -> (12.4201, -22.0715) centre (6.2201, -22.0709) ccw
  line L7 (12.4201, -14.7709) -> (12.4201, -22.0715)
  arc A16 (12.4201, -14.7709) -> (6.2201, -8.5709) centre (6.2201, -14.7709) ccw
  line L8 (-6.2799, -8.5709) -> (6.2201, -8.5709)
  line L9 (8.9318, -27.6464) -> (8.5863, -26.8133)
  line L10 (4.1692, -29.2709) -> (4.0199, -28.3709)
  line L11 (-4.2289, -29.2709) -> (-4.0796, -28.3709)
  line L12 (-8.6461, -26.8133) -> (-8.9915, -27.6464)
  line L13 (-12.4799, -22.0715) -> (-12.4799, -14.7709)
  line L14 (-11.5799, -14.7709) -> (-11.5799, -22.0715)
  line L15 (-11.2799, -22.0715) -> (-11.2799, -14.7709)
  dimension "d186" = 1
  constraint coincident A5.start L2.start
  constraint coincident A8.end L2.end
  constraint concentric A5 A9
  constraint concentric A8 A10
  constraint concentric A7 A11
  constraint concentric A6 A12
  constraint tangent L3 A12
  constraint tangent L3 A9
  constraint concentric A6 A13
  constraint concentric A7 A14
  constraint concentric A8 A15
  constraint concentric A5 A16
  constraint tangent A13 L8
  constraint tangent A16 L8
  constraint tangent A13 L13
  constraint parallel L13 L14
  constraint coincident A7.start L15.start
  constraint coincident A6.end L15.end
extrude "Extrude40" cut sketch "Sketch32" against normal blind 1 contours A3 | A4 bodies 6
sketch "Sketch33" plane through (0, 0, 140.75) normal (0, 0, 1) x (-1, 0, 0)
  line L0 (-0.0497, -5.8) -> (-16.5023, -7.1657)
  line L1 (-16.5023, -7.1657) -> (-16.403, -8.3615)
  line L2 (-16.403, -8.3615) -> (-11.4201, -7.9479)
  line L3 (-11.4201, -7.9479) -> (0, -7)
  line L4 (0, -7) -> (11.4799, -7)
  line L5 (11.4799, -7) -> (17, -7)
  line L6 (17, -7) -> (17, -5.8)
  line L7 (17, -5.8) -> (11.4799, -5.8)
  line L8 (11.4799, -5.8) -> (-0.0497, -5.8)
  line L9 (4.4828, -7) -> (4.4828, -5.8)
  line L10 (-4.4658, -7.3707) -> (-4.5651, -6.1748)
  constraint coincident L4 L9.start
  constraint coincident L8 L9.end
  constraint perpendicular L8 L9
  constraint coincident L3 L10.start
  constraint coincident L0 L10.end
  constraint perpendicular L0 L10
extrude "Extrude41" add sketch "Sketch33" along normal blind 18 contours L0 L1 L2 L3 L10 | L4 L5 L6 L7 L8 L9 bodies 2
extrude "Extrude42" add sketch "Sketch32" along normal blind 17.5 contours L3 A9 L4 A10 A11 A12 A13 A14 A15 L7 A16 L8 L9 L12 L13 L14 | L5 L6 L10 L11 bodies 6